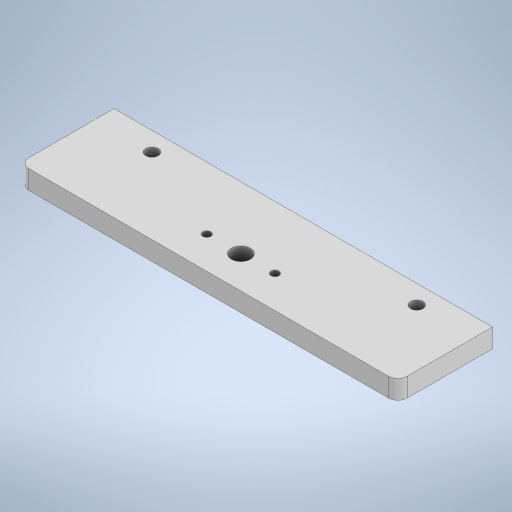
# Autodesk Inventor part: Nap_duoi
Saved by Autodesk Inventor 2023 (Build 270158000, 158)
## iProperties
Created: 2025-04-07
Part Number: Nap_duoi
Material: Generic
Document SubType Name: Modeling
Designer: huyqu
Density: 1 g/cm^3
Appearance: Default
Author: huyqu
Autodesk Inventor part; units mm, degrees
ref_plane "YZ Plane" through (0, 0, 0) normal (1, 0, 0) x (0, 1, 0)
ref_plane "XZ Plane" through (0, 0, 0) normal (0, 1, 0) x (-1, 0, 0)
ref_plane "XY Plane" through (0, 0, 0) normal (0, 0, 1) x (1, 0, 0)
sketch "Sketch1" plane through (0, 0, 0) normal (0, 0, 1) x (1, 0, 0)
  line L0 (0, 0) -> (200, 0)
  line L1 (200, 0) -> (200, 10)
  line L2 (200, 10) -> (0, 10)
  line L3 (0, 10) -> (0, 0)
  dimension "d0" = 200
  dimension "d1" = 10
  constraints: 8 end point, 2 parallel, 1 horizontal, 1 perpendicular
  measures "d0" distance of L1.end L2.end
  measures "d1" distance of L0.end L1.end
extrude "Extrusion1" add sketch "Sketch1" along normal blind 50
sketch "Sketch2" plane through (0, 10, 0) normal (0, 1, 0) x (1, 0, 0)
  line L0 (200, 0) -> (200, -50) projected
  line L1 (200, -23) -> (-0.0003, -23)
  line L2 (200, 0) -> (0, 0) projected
  line L3 (100, 0) -> (100, -50)
  line L4 (200, -50) -> (0, -50) projected
  circle A0 centre (81.9998, -23) radius 2.5
  circle A1 centre (117.9998, -23) radius 2.5
  point P0 (99.9998, -23)
  dimension "d4" = 23
  dimension "d5" = 5
  dimension "d6" = 5
  dimension "d7" = 18
  dimension "d8" = 36
  constraints: 4 end point, 3 midpoint, 3 point on line, 2 centre point, 1 perpendicular
  measures "d4" distance between parallel lines of L1 L2
  measures "d5" diameter of A0
  measures "d6" diameter of A1
  measures "d7" distance of point (100, -23) A0.centre
  measures "d8" distance of A1.centre A0.centre
sketch "Sketch3" plane through (0, 0, 0) normal (0, 0, -1) x (-1, 0, 0)
  line L0 (0, 0) -> (-200, 0) projected
  line L1 (-200, 10) -> (0, 10) projected
  line L2 (0, 0) -> (-200, 0)
  line L3 (-200, 0) -> (-200, 10)
  line L4 (-200, 10) -> (0, 10)
  line L5 (0, 10) -> (0, 0)
  constraints: 8 end point, 2 parallel, 1 horizontal, 1 perpendicular
extrude "Extrusion3" add sketch "Sketch3" along normal blind 10
sketch "Sketch4" plane through (0, 10, 50) normal (0, 1, 0) x (1, 0, 0)
  line L0 (0, 0) -> (200, 0) projected
  line L1 (100, 0) -> (100, 60)
  line L2 (0, 60) -> (200, 60) projected
  circle A0 centre (100, 27) radius 5
  point P0 (0, 50)
  dimension "d17" = 10
  dimension "d39" = 33
  constraints: 2 end point, 2 midpoint, 1 centre point, 1 point on line
  measures "d17" diameter of A0
  measures "d39" distance from line of L2 A0.centre
extrude "Extrusion4" cut sketch "Sketch4" against normal blind 10
sketch "Sketch5" plane through (0, 0, 50) normal (0, -1, 0) x (1, 0, 0)
  line L0 (140, -40) -> (140, -50) projected
  line L1 (140, -50) -> (60, -50) projected
  line L2 (60, -50) -> (60, -40) projected
  line L3 (0, -40) -> (60, -40) projected
  line L4 (0, -60) -> (0, -40) projected
  line L5 (0, -60) -> (200, -60) projected
  line L6 (200, -60) -> (200, -40) projected
  line L7 (140, -40) -> (200, -40) projected
  circle A0 centre (30, -50) radius 2.4585 projected
  circle A1 centre (170, -50) radius 2.4585 projected
  point P0 (0, -50)
  point P1 (170, -50)
  point P2 (30, -50)
  point P3 (200, -50)
  point P4 (170, -40)
  point P5 (30, -40)
  constraints: 3 midpoint, 2 horizontal alignment, 2 vertical alignment
hole "Hole1" at (170, 0, 0) at (30, 0, 0) direction (0, 1, 0) diameter 6.5 end through all counterbore diameter 11 counterbore depth 5
hole "Hole2" at (81.9998, 10, 23) at (117.9998, 10, 23) direction (0, -1, 0) diameter 4.134 end through all thread size "M5x0.8" class "6H" standard "ISO Metric profile"
sketch "Sketch6" plane through (0, 10, 50) normal (0, 1, 0) x (1, 0, 0)
  line L0 (200, 0) -> (0, 0) projected
  line L1 (0, 0) -> (200, 0)
  line L2 (200, 0) -> (200, 10)
  line L3 (200, 10) -> (0, 10)
  line L4 (0, 10) -> (0, 0)
  point P0 (0, 50)
  dimension "d35" = 10
  constraints: 8 end point, 2 parallel, 1 horizontal, 1 perpendicular
  measures "d35" distance between parallel lines of L3 L0
extrude "Extrusion5" cut sketch "Sketch6" against normal through all
sketch "Sketch7" plane through (0, 10, -10) normal (0, 1, 0) x (1, 0, 0)
  point P0 (0, -10)
fillet "Fillet3" radius 5 2 edges at (0, 5, 40) (200, 5, 40)
body "Solid1"
